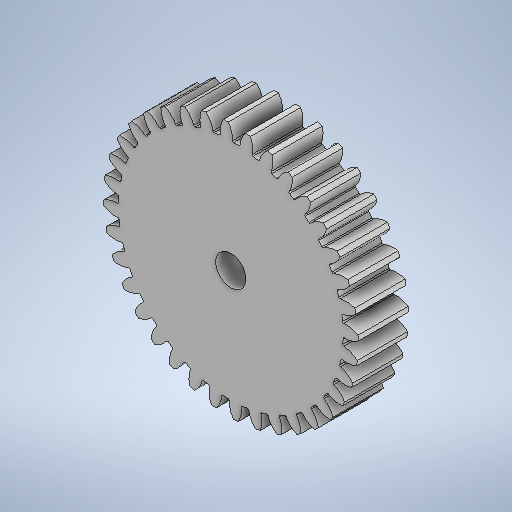
# Autodesk Inventor part: Gear36
Saved by Autodesk Inventor 2025.1 (Build 291241000, 241)
## iProperties
Created: 2024-11-04
Part Number: Gear36
Material: Generic
Document SubType Name: Modeling
Designer: rishi
Density: 1 g/cm^3
Appearance: Default
Author: rishi
Autodesk Inventor part; units mm, degrees
ref_plane "YZ Plane" through (0, 0, 0) normal (1, 0, 0) x (0, 1, 0)
ref_plane "XZ Plane" through (0, 0, 0) normal (0, 1, 0) x (-1, 0, 0)
ref_plane "XY Plane" through (0, 0, 0) normal (0, 0, 1) x (1, 0, 0)
sketch "Sketch1" plane through (0, 0, 0) normal (0, 0, 1) x (1, 0, 0)
  circle A0 centre (0, 0) radius 33.5
  arc A1 (0.5306, 33.8247) -> (-0.7651, 37.9923) centre (-6.466, 33.9346) ccw
  line L0 (-12.932, 31.2595) -> (-12.9324, 31.2593)
  arc A2 (-2.2265, 37.9347) -> (-3.1904, 33.6781) centre (3.7759, 34.3381) ccw
  arc A3 (0.5306, 33.8247) -> (0.8511, 33.4892) centre (0.8595, 33.818) ccw
  arc A4 (-3.4834, 33.3184) -> (-3.1904, 33.6781) centre (-3.5176, 33.6455) ccw
  arc A5 (-0.7651, 37.9923) -> (-2.2265, 37.9347) centre (0, 0) ccw
  arc A6 (-8.78, 36.9718) -> (-8.99, 32.6125) centre (-2.2442, 34.4722) ccw
  arc A7 (-7.3508, 37.2822) -> (-8.78, 36.9718) centre (0, 0) ccw
  arc A8 (-5.351, 33.403) -> (-7.3508, 37.2822) centre (-12.2604, 32.2963) ccw
  arc A9 (-5.351, 33.403) -> (-4.9771, 33.1282) centre (-5.026, 33.4535) ccw
  arc A10 (-9.2162, 32.2073) -> (-8.99, 32.6125) centre (-9.3067, 32.5235) ccw
  arc A11 (-15.0667, 34.8854) -> (-14.5166, 30.5559) centre (-8.1961, 33.5588) ccw
  arc A12 (-13.7131, 35.4394) -> (-15.0667, 34.8854) centre (0, 0) ccw
  arc A13 (-11.0701, 31.9663) -> (-13.7131, 35.4394) centre (-17.6824, 29.6766) ccw
  arc A14 (-11.0701, 31.9663) -> (-10.6542, 31.7606) centre (-10.7588, 32.0725) ccw
  arc A15 (-14.6689, 30.1176) -> (-14.5166, 30.5559) centre (-14.8129, 30.4133) ccw
  arc A16 (-20.8956, 31.7392) -> (-19.602, 27.5709) centre (-13.899, 31.6257) ccw
  arc A17 (-19.6587, 32.5197) -> (-20.8956, 31.7392) centre (0, 0) ccw
  arc A18 (-16.4528, 29.5584) -> (-19.6587, 32.5197) centre (-22.567, 26.1552) ccw
  arc A19 (-16.4528, 29.5584) -> (-16.0075, 29.428) centre (-16.1647, 29.717) ccw
  arc A20 (-19.676, 27.1129) -> (-19.602, 27.5709) centre (-19.8691, 27.379) ccw
  arc A21 (-26.0896, 27.6285) -> (-24.0918, 23.7482) centre (-19.1796, 28.7317) ccw
  arc A22 (-25.0071, 28.612) -> (-26.0896, 27.6285) centre (0, 0) ccw
  arc A23 (-21.3356, 26.2523) -> (-25.0071, 28.612) centre (-26.766, 21.8392) ccw
  arc A24 (-21.3356, 26.2523) -> (-20.8744, 26.2013) centre (-21.0794, 26.4585) ccw
  arc A25 (-24.0851, 23.2843) -> (-24.0918, 23.7482) centre (-24.3216, 23.5129) ccw
  arc A26 (-30.4909, 22.6783) -> (-27.8497, 19.2039) centre (-23.8774, 24.9647) ccw
  arc A27 (-29.5956, 23.8349) -> (-30.4909, 22.6783) centre (0, 0) ccw
  arc A28 (-25.5702, 22.1486) -> (-29.5956, 23.8349) centre (-30.1517, 16.8595) ccw
  arc A29 (-25.5702, 22.1486) -> (-25.1071, 22.1784) centre (-25.3536, 22.3962) ccw
  arc A30 (-27.7625, 18.7482) -> (-27.8497, 19.2039) centre (-28.0351, 18.9322) ccw
  arc A31 (-33.9657, 17.0391) -> (-30.7613, 14.0761) centre (-27.8497, 20.4391) ccw
  arc A32 (-33.2848, 18.3336) -> (-33.9657, 17.0391) centre (0, 0) ccw
  arc A33 (-29.0278, 17.3719) -> (-33.2848, 18.3336) centre (-32.6212, 11.3676) ccw
  arc A34 (-29.0278, 17.3719) -> (-28.5769, 17.4817) centre (-28.8575, 17.6533) ccw
  arc A35 (-30.5963, 13.6424) -> (-30.7613, 14.0761) centre (-30.8967, 13.7764) ccw
  arc A36 (-36.4085, 10.8822) -> (-32.7383, 8.5206) centre (-30.9759, 15.2926) ccw
  arc A37 (-35.9628, 12.2752) -> (-36.4085, 10.8822) centre (0, 0) ccw
  arc A38 (-31.6034, 12.0674) -> (-35.9628, 12.2752) centre (-34.0996, 5.5303) ccw
  arc A39 (-31.6034, 12.0674) -> (-31.1784, 12.2538) centre (-31.4845, 12.3741) ccw
  arc A40 (-32.5005, 8.1222) -> (-32.7383, 8.5206) centre (-32.8195, 8.2019) ccw
  arc A41 (-37.745, 4.3946) -> (-33.7205, 2.7062) centre (-33.1608, 9.6813) ccw
  arc A42 (-37.548, 5.8438) -> (-37.745, 4.3946) centre (0, 0) ccw
  arc A43 (-33.2187, 6.3962) -> (-37.548, 5.8438) centre (-34.5419, -0.4751) ccw
  arc A44 (-33.2187, 6.3962) -> (-32.8326, 6.6535) centre (-33.155, 6.7189) ccw
  arc A45 (-33.4171, 2.3552) -> (-33.7205, 2.7062) centre (-33.7452, 2.3783) ccw
  arc A46 (-37.9347, -2.2265) -> (-33.6781, -3.1904) centre (-34.3381, 3.7759) ccw
  arc A47 (-37.9923, -0.7651) -> (-37.9347, -2.2265) centre (0, 0) ccw
  arc A48 (-33.8247, 0.5306) -> (-37.9923, -0.7651) centre (-33.9346, -6.466) ccw
  arc A49 (-33.8247, 0.5306) -> (-33.4892, 0.8511) centre (-33.818, 0.8595) ccw
  arc A50 (-33.3184, -3.4834) -> (-33.6781, -3.1904) centre (-33.6455, -3.5176) ccw
  arc A51 (-36.9718, -8.78) -> (-32.6125, -8.99) centre (-34.4722, -2.2442) ccw
  arc A52 (-37.2822, -7.3508) -> (-36.9718, -8.78) centre (0, 0) ccw
  arc A53 (-33.403, -5.351) -> (-37.2822, -7.3508) centre (-32.2963, -12.2604) ccw
  arc A54 (-33.403, -5.351) -> (-33.1282, -4.9771) centre (-33.4535, -5.026) ccw
  arc A55 (-32.2073, -9.2162) -> (-32.6125, -8.99) centre (-32.5235, -9.3067) ccw
  arc A56 (-34.8854, -15.0667) -> (-30.5559, -14.5166) centre (-33.5588, -8.1961) ccw
  arc A57 (-35.4394, -13.7131) -> (-34.8854, -15.0667) centre (0, 0) ccw
  arc A58 (-31.9663, -11.0701) -> (-35.4394, -13.7131) centre (-29.6766, -17.6824) ccw
  arc A59 (-31.9663, -11.0701) -> (-31.7606, -10.6542) centre (-32.0725, -10.7588) ccw
  arc A60 (-30.1176, -14.6689) -> (-30.5559, -14.5166) centre (-30.4133, -14.8129) ccw
  arc A61 (-31.7392, -20.8956) -> (-27.5709, -19.602) centre (-31.6257, -13.899) ccw
  arc A62 (-32.5197, -19.6587) -> (-31.7392, -20.8956) centre (0, 0) ccw
  arc A63 (-29.5584, -16.4528) -> (-32.5197, -19.6587) centre (-26.1552, -22.567) ccw
  arc A64 (-29.5584, -16.4528) -> (-29.428, -16.0075) centre (-29.717, -16.1647) ccw
  arc A65 (-27.1129, -19.676) -> (-27.5709, -19.602) centre (-27.379, -19.8691) ccw
  arc A66 (-27.6285, -26.0896) -> (-23.7482, -24.0918) centre (-28.7317, -19.1796) ccw
  arc A67 (-28.612, -25.0071) -> (-27.6285, -26.0896) centre (0, 0) ccw
  arc A68 (-26.2523, -21.3356) -> (-28.612, -25.0071) centre (-21.8392, -26.766) ccw
  arc A69 (-26.2523, -21.3356) -> (-26.2013, -20.8744) centre (-26.4585, -21.0794) ccw
  arc A70 (-23.2843, -24.0851) -> (-23.7482, -24.0918) centre (-23.5129, -24.3216) ccw
  arc A71 (-22.6783, -30.4909) -> (-19.2039, -27.8497) centre (-24.9647, -23.8774) ccw
  arc A72 (-23.8349, -29.5956) -> (-22.6783, -30.4909) centre (0, 0) ccw
  arc A73 (-22.1486, -25.5702) -> (-23.8349, -29.5956) centre (-16.8595, -30.1517) ccw
  arc A74 (-22.1486, -25.5702) -> (-22.1784, -25.1071) centre (-22.3962, -25.3536) ccw
  arc A75 (-18.7482, -27.7625) -> (-19.2039, -27.8497) centre (-18.9322, -28.0351) ccw
  arc A76 (-17.0391, -33.9657) -> (-14.0761, -30.7613) centre (-20.4391, -27.8497) ccw
  arc A77 (-18.3336, -33.2848) -> (-17.0391, -33.9657) centre (0, 0) ccw
  arc A78 (-17.3719, -29.0278) -> (-18.3336, -33.2848) centre (-11.3676, -32.6212) ccw
  arc A79 (-17.3719, -29.0278) -> (-17.4817, -28.5769) centre (-17.6533, -28.8575) ccw
  arc A80 (-13.6424, -30.5963) -> (-14.0761, -30.7613) centre (-13.7764, -30.8967) ccw
  arc A81 (-10.8822, -36.4085) -> (-8.5206, -32.7383) centre (-15.2926, -30.9759) ccw
  arc A82 (-12.2752, -35.9628) -> (-10.8822, -36.4085) centre (0, 0) ccw
  arc A83 (-12.0674, -31.6034) -> (-12.2752, -35.9628) centre (-5.5303, -34.0996) ccw
  arc A84 (-12.0674, -31.6034) -> (-12.2538, -31.1784) centre (-12.3741, -31.4845) ccw
  arc A85 (-8.1222, -32.5005) -> (-8.5206, -32.7383) centre (-8.2019, -32.8195) ccw
  arc A86 (-4.3946, -37.745) -> (-2.7062, -33.7205) centre (-9.6813, -33.1608) ccw
  arc A87 (-5.8438, -37.548) -> (-4.3946, -37.745) centre (0, 0) ccw
  arc A88 (-6.3962, -33.2187) -> (-5.8438, -37.548) centre (0.4751, -34.5419) ccw
  arc A89 (-6.3962, -33.2187) -> (-6.6535, -32.8326) centre (-6.7189, -33.155) ccw
  arc A90 (-2.3552, -33.4171) -> (-2.7062, -33.7205) centre (-2.3783, -33.7452) ccw
  arc A91 (2.2265, -37.9347) -> (3.1904, -33.6781) centre (-3.7759, -34.3381) ccw
  arc A92 (0.7651, -37.9923) -> (2.2265, -37.9347) centre (0, 0) ccw
  arc A93 (-0.5306, -33.8247) -> (0.7651, -37.9923) centre (6.466, -33.9346) ccw
  arc A94 (-0.5306, -33.8247) -> (-0.8511, -33.4892) centre (-0.8595, -33.818) ccw
  arc A95 (3.4834, -33.3184) -> (3.1904, -33.6781) centre (3.5176, -33.6455) ccw
  arc A96 (8.78, -36.9718) -> (8.99, -32.6125) centre (2.2442, -34.4722) ccw
  arc A97 (7.3508, -37.2822) -> (8.78, -36.9718) centre (0, 0) ccw
  arc A98 (5.351, -33.403) -> (7.3508, -37.2822) centre (12.2604, -32.2963) ccw
  arc A99 (5.351, -33.403) -> (4.9771, -33.1282) centre (5.026, -33.4535) ccw
  arc A100 (9.2162, -32.2073) -> (8.99, -32.6125) centre (9.3067, -32.5235) ccw
  arc A101 (15.0667, -34.8854) -> (14.5166, -30.5559) centre (8.1961, -33.5588) ccw
  arc A102 (13.7131, -35.4394) -> (15.0667, -34.8854) centre (0, 0) ccw
  arc A103 (11.0701, -31.9663) -> (13.7131, -35.4394) centre (17.6824, -29.6766) ccw
  arc A104 (11.0701, -31.9663) -> (10.6542, -31.7606) centre (10.7588, -32.0725) ccw
  arc A105 (14.6689, -30.1176) -> (14.5166, -30.5559) centre (14.8129, -30.4133) ccw
  arc A106 (20.8956, -31.7392) -> (19.602, -27.5709) centre (13.899, -31.6257) ccw
  arc A107 (19.6587, -32.5197) -> (20.8956, -31.7392) centre (0, 0) ccw
  arc A108 (16.4528, -29.5584) -> (19.6587, -32.5197) centre (22.567, -26.1552) ccw
  arc A109 (16.4528, -29.5584) -> (16.0075, -29.428) centre (16.1647, -29.717) ccw
  arc A110 (19.676, -27.1129) -> (19.602, -27.5709) centre (19.8691, -27.379) ccw
  arc A111 (26.0896, -27.6285) -> (24.0918, -23.7482) centre (19.1796, -28.7317) ccw
  arc A112 (25.0071, -28.612) -> (26.0896, -27.6285) centre (0, 0) ccw
  arc A113 (21.3356, -26.2523) -> (25.0071, -28.612) centre (26.766, -21.8392) ccw
  arc A114 (21.3356, -26.2523) -> (20.8744, -26.2013) centre (21.0794, -26.4585) ccw
  arc A115 (24.0851, -23.2843) -> (24.0918, -23.7482) centre (24.3216, -23.5129) ccw
  arc A116 (30.4909, -22.6783) -> (27.8497, -19.2039) centre (23.8774, -24.9647) ccw
  arc A117 (29.5956, -23.8349) -> (30.4909, -22.6783) centre (0, 0) ccw
  arc A118 (25.5702, -22.1486) -> (29.5956, -23.8349) centre (30.1517, -16.8595) ccw
  arc A119 (25.5702, -22.1486) -> (25.1071, -22.1784) centre (25.3536, -22.3962) ccw
  arc A120 (27.7625, -18.7482) -> (27.8497, -19.2039) centre (28.0351, -18.9322) ccw
  arc A121 (33.9657, -17.0391) -> (30.7613, -14.0761) centre (27.8497, -20.4391) ccw
  arc A122 (33.2848, -18.3336) -> (33.9657, -17.0391) centre (0, 0) ccw
  arc A123 (29.0278, -17.3719) -> (33.2848, -18.3336) centre (32.6212, -11.3676) ccw
  arc A124 (29.0278, -17.3719) -> (28.5769, -17.4817) centre (28.8575, -17.6533) ccw
  arc A125 (30.5963, -13.6424) -> (30.7613, -14.0761) centre (30.8967, -13.7764) ccw
  arc A126 (36.4085, -10.8822) -> (32.7383, -8.5206) centre (30.9759, -15.2926) ccw
  arc A127 (35.9628, -12.2752) -> (36.4085, -10.8822) centre (0, 0) ccw
  arc A128 (31.6034, -12.0674) -> (35.9628, -12.2752) centre (34.0996, -5.5303) ccw
  arc A129 (31.6034, -12.0674) -> (31.1784, -12.2538) centre (31.4845, -12.3741) ccw
  arc A130 (32.5005, -8.1222) -> (32.7383, -8.5206) centre (32.8195, -8.2019) ccw
  arc A131 (37.745, -4.3946) -> (33.7205, -2.7062) centre (33.1608, -9.6813) ccw
  arc A132 (37.548, -5.8438) -> (37.745, -4.3946) centre (0, 0) ccw
  arc A133 (33.2187, -6.3962) -> (37.548, -5.8438) centre (34.5419, 0.4751) ccw
  arc A134 (33.2187, -6.3962) -> (32.8326, -6.6535) centre (33.155, -6.7189) ccw
  arc A135 (33.4171, -2.3552) -> (33.7205, -2.7062) centre (33.7452, -2.3783) ccw
  arc A136 (37.9347, 2.2265) -> (33.6781, 3.1904) centre (34.3381, -3.7759) ccw
  arc A137 (37.9923, 0.7651) -> (37.9347, 2.2265) centre (0, 0) ccw
  arc A138 (33.8247, -0.5306) -> (37.9923, 0.7651) centre (33.9346, 6.466) ccw
  arc A139 (33.8247, -0.5306) -> (33.4892, -0.8511) centre (33.818, -0.8595) ccw
  arc A140 (33.3184, 3.4834) -> (33.6781, 3.1904) centre (33.6455, 3.5176) ccw
  arc A141 (36.9718, 8.78) -> (32.6125, 8.99) centre (34.4722, 2.2442) ccw
  arc A142 (37.2822, 7.3508) -> (36.9718, 8.78) centre (0, 0) ccw
  arc A143 (33.403, 5.351) -> (37.2822, 7.3508) centre (32.2963, 12.2604) ccw
  arc A144 (33.403, 5.351) -> (33.1282, 4.9771) centre (33.4535, 5.026) ccw
  arc A145 (32.2073, 9.2162) -> (32.6125, 8.99) centre (32.5235, 9.3067) ccw
  arc A146 (34.8854, 15.0667) -> (30.5559, 14.5166) centre (33.5588, 8.1961) ccw
  arc A147 (35.4394, 13.7131) -> (34.8854, 15.0667) centre (0, 0) ccw
  arc A148 (31.9663, 11.0701) -> (35.4394, 13.7131) centre (29.6766, 17.6824) ccw
  arc A149 (31.9663, 11.0701) -> (31.7606, 10.6542) centre (32.0725, 10.7588) ccw
  arc A150 (30.1176, 14.6689) -> (30.5559, 14.5166) centre (30.4133, 14.8129) ccw
  arc A151 (31.7392, 20.8956) -> (27.5709, 19.602) centre (31.6257, 13.899) ccw
  arc A152 (32.5197, 19.6587) -> (31.7392, 20.8956) centre (0, 0) ccw
  arc A153 (29.5584, 16.4528) -> (32.5197, 19.6587) centre (26.1552, 22.567) ccw
  arc A154 (29.5584, 16.4528) -> (29.428, 16.0075) centre (29.717, 16.1647) ccw
  arc A155 (27.1129, 19.676) -> (27.5709, 19.602) centre (27.379, 19.8691) ccw
  arc A156 (27.6285, 26.0896) -> (23.7482, 24.0918) centre (28.7317, 19.1796) ccw
  arc A157 (28.612, 25.0071) -> (27.6285, 26.0896) centre (0, 0) ccw
  arc A158 (26.2523, 21.3356) -> (28.612, 25.0071) centre (21.8392, 26.766) ccw
  arc A159 (26.2523, 21.3356) -> (26.2013, 20.8744) centre (26.4585, 21.0794) ccw
  arc A160 (23.2843, 24.0851) -> (23.7482, 24.0918) centre (23.5129, 24.3216) ccw
  arc A161 (22.6783, 30.4909) -> (19.2039, 27.8497) centre (24.9647, 23.8774) ccw
  arc A162 (23.8349, 29.5956) -> (22.6783, 30.4909) centre (0, 0) ccw
  arc A163 (22.1486, 25.5702) -> (23.8349, 29.5956) centre (16.8595, 30.1517) ccw
  arc A164 (22.1486, 25.5702) -> (22.1784, 25.1071) centre (22.3962, 25.3536) ccw
  arc A165 (18.7482, 27.7625) -> (19.2039, 27.8497) centre (18.9322, 28.0351) ccw
  arc A166 (17.0391, 33.9657) -> (14.0761, 30.7613) centre (20.4391, 27.8497) ccw
  arc A167 (18.3336, 33.2848) -> (17.0391, 33.9657) centre (0, 0) ccw
  arc A168 (17.3719, 29.0278) -> (18.3336, 33.2848) centre (11.3676, 32.6212) ccw
  arc A169 (17.3719, 29.0278) -> (17.4817, 28.5769) centre (17.6533, 28.8575) ccw
  arc A170 (13.6424, 30.5963) -> (14.0761, 30.7613) centre (13.7764, 30.8967) ccw
  arc A171 (10.8822, 36.4085) -> (8.5206, 32.7383) centre (15.2926, 30.9759) ccw
  arc A172 (12.2752, 35.9628) -> (10.8822, 36.4085) centre (0, 0) ccw
  arc A173 (12.0674, 31.6034) -> (12.2752, 35.9628) centre (5.5303, 34.0996) ccw
  arc A174 (12.0674, 31.6034) -> (12.2538, 31.1784) centre (12.3741, 31.4845) ccw
  arc A175 (8.1222, 32.5005) -> (8.5206, 32.7383) centre (8.2019, 32.8195) ccw
  arc A176 (4.3946, 37.745) -> (2.7062, 33.7205) centre (9.6813, 33.1608) ccw
  arc A177 (5.8438, 37.548) -> (4.3946, 37.745) centre (0, 0) ccw
  arc A178 (6.3962, 33.2187) -> (5.8438, 37.548) centre (-0.4751, 34.5419) ccw
  arc A179 (6.3962, 33.2187) -> (6.6535, 32.8326) centre (6.7189, 33.155) ccw
  arc A180 (2.3552, 33.4171) -> (2.7062, 33.7205) centre (2.3783, 33.7452) ccw
  point P0 (-19.676, 27.1129)
  point P1 (-20.8744, 26.2013)
  point P2 (-24.0851, 23.2843)
  point P3 (-25.1071, 22.1784)
  point P4 (-27.7625, 18.7482)
  point P5 (-28.5769, 17.4817)
  point P6 (-33.1282, -4.9771)
  point P7 (-32.2073, -9.2162)
  point P8 (-31.7606, -10.6542)
  point P9 (-29.428, -16.0075)
  point P10 (-27.1129, -19.676)
  point P11 (-26.2013, -20.8744)
  point P12 (-22.1784, -25.1071)
  point P13 (-18.7482, -27.7625)
  point P14 (-17.4817, -28.5769)
  point P15 (-13.6424, -30.5963)
  point P16 (14.6689, -30.1176)
  point P17 (20.8744, -26.2013)
  point P18 (24.0851, -23.2843)
  point P19 (25.1071, -22.1784)
  point P20 (27.7625, -18.7482)
  point P21 (33.1282, 4.9771)
  point P22 (26.2013, 20.8744)
  point P23 (22.1784, 25.1071)
  point P24 (12.2538, 31.1784)
  point P25 (-4.9771, 33.1282)
  point P26 (-9.2162, 32.2073)
  point P27 (-10.6542, 31.7606)
  dimension "d14" = 360
  constraints: 360 point on circle, 180 centre point, 2 end point, 1 coincident, 582 other
extrude "Extrusion1" add sketch "Sketch1" along normal blind 15
sketch "Sketch2" plane through (0, 0, 15) normal (0, 0, 1) x (1, 0, 0)
  circle A0 centre (0, 0) radius 4.5
  dimension "d18" = 9
  constraints: 1 centre point, 1 coincident
  measures "d18" diameter of A0
extrude "Extrusion2" cut sketch "Sketch2" against normal blind 15
body "Solid1"
